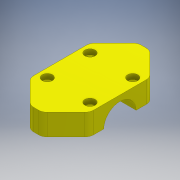
# Autodesk Inventor part: Y Carriage Clamp 1.0
Saved by Autodesk Inventor 2016 (Build 200138000, 138)
## iProperties
Created: 2017-02-14
Part Number: Y Carriage Clamp 1.0
Material: PC/ABS Plastic
Document SubType Name: Modeling
Designer: Scott
Density: 0.357273 g/cm^3
Appearance: Smooth - Yellow
Author: Scott
## iProperties of the stored document Y Carriage Clamp 1.0_3DPrint.ipt
Created: 2017-04-11
Part Number: Y Carriage Clamp 1.0_3DPrint
Material: Generic
Document SubType Name: Modeling
Designer: Scott
Density: 1 g/cm^3
Appearance: Default
Author: Scott
Autodesk Inventor part; units mm, degrees
ref_plane "YZ Plane" through (0, 0, 0) normal (1, 0, 0) x (0, 1, 0)
ref_plane "XZ Plane" through (0, 0, 0) normal (0, 1, 0) x (-1, 0, 0)
ref_plane "XY Plane" through (0, 0, 0) normal (0, 0, 1) x (1, 0, 0)
sketch "Sketch1" plane through (0, 0, 0) normal (0, 0, 1) x (1, 0, 0)
  line L0 (0, 0) -> (0, 37.7883) construction
  line L1 (0, 0) -> (33.2061, 0) construction
  line L2 (-17.5, 16.5) -> (17.5, 16.5)
  line L3 (17.5, 16.5) -> (17.5, -16.5)
  line L4 (17.5, -16.5) -> (-17.5, -16.5)
  line L5 (-17.5, -16.5) -> (-17.5, 16.5)
  line L6 (-17.5, 16.5) -> (-17.5, 17.5)
  line L7 (-17.5, 17.5) -> (-3.5, 31.5)
  line L8 (-3.5, 31.5) -> (3.5, 31.5)
  line L9 (3.5, 31.5) -> (17.5, 17.5)
  line L10 (17.5, 17.5) -> (17.5, 16.5)
  line L11 (-17.5, -16.5) -> (17.5, -16.5)
  line L12 (-17.5, -16.5) -> (-17.5, -17.5)
  line L13 (-17.5, -17.5) -> (-3.5, -31.5)
  line L14 (-3.5, -31.5) -> (3.5, -31.5)
  line L15 (3.5, -31.5) -> (17.5, -17.5)
  line L16 (17.5, -17.5) -> (17.5, -16.5)
  point P0 (0, 16.5)
  point P1 (17.5, 0)
  point P2 (0, -16.5)
  dimension "d0" = 35
  dimension "d1" = 33
  dimension "d2" = 1
  dimension "d3" = 1
  dimension "d4" = 45
  dimension "d5" = 45
  dimension "d6" = 31.5
  constraints: 34 end point, 5 symmetric about line, 3 parallel, 2 horizontal, 2 midpoint, 2 perpendicular, 2 point on line, 2 vertical
  measures "d0" distance of L2.start L2.end
  measures "d1" distance of L2.end L3.end
  measures "d2" distance from line of L2 L9.end
  measures "d3" distance of L2.start L6.end
  measures "d4" angle of L7 L2
  measures "d5" angle of L2 L9
  measures "d6" distance between parallel lines of L8 L1
extrude "Extrusion1" add sketch "Sketch1" along normal blind 12.5
sketch "Sketch2" plane through (17.5, -17.5, 0) normal (1, 0, 0) x (0, 0, -1)
  line L0 (0, 17.5) -> (18.5906, 17.5) construction
  circle A0 centre (0.25, 17.5) radius 9.5
  dimension "d9" = 0.25
  dimension "d10" = 19
  constraints: 2 end point, 1 centre point, 1 horizontal, 1 point on line
  measures "d9" distance of L0.start A0.centre
  measures "d10" diameter of A0
extrude "Extrusion2" cut sketch "Sketch2" against normal through all
sketch "Sketch3" plane through (0, 0, 12.5) normal (0, 0, 1) x (1, 0, 0)
  line L0 (0, 0) -> (23.8971, 0) construction
  line L1 (0, 0) -> (0, 42.5414) construction
  line L2 (-12.5, 12.5) -> (12.5, 12.5) construction
  line L3 (12.5, 12.5) -> (12.5, -12.5) construction
  line L4 (12.5, -12.5) -> (-12.5, -12.5) construction
  line L5 (-12.5, -12.5) -> (-12.5, 12.5) construction
  point P0 (12.5, 0)
  point P1 (0, 12.5)
  dimension "d13" = 25
  dimension "d14" = 25
  constraints: 12 end point, 4 coincident, 2 horizontal, 2 midpoint, 2 parallel, 2 point on line, 1 perpendicular, 1 vertical
  measures "d13" distance of L2.end L3.end
  measures "d14" distance of L2.start L2.end
hole "Hole1" at (-12.5, 12.5, 12.5) at (-12.5, -12.5, 12.5) at (12.5, -12.5, 12.5) at (12.5, 12.5, 12.5) direction (0, 0, -1) diameter 3.5 end through all counterbore diameter 6 counterbore depth 3
fillet "Fillet1" radius 5 8 edges at (3.5, 31.5, 6.25) (-3.5, 31.5, 6.25) (-17.5, 17.5, 6.25) (17.5, 17.5, 6.25) (-17.5, -17.5, 6.25) (-3.5, -31.5, 6.25) (3.5, -31.5, 6.25) (17.5, -17.5, 6.25)
sketch "Sketch4" plane through (0, 0, 0) normal (0, 0, -1) x (-1, 0, 0)
  line L0 (0, 0) -> (0, 38.8983) construction
  line L1 (0, 0) -> (0, -39.4176) construction
  circle A0 centre (0, 22.5) radius 5.5
  circle A1 centre (0, -22.5) radius 5.5
  dimension "d23" = 11
  dimension "d24" = 22.5
  dimension "d25" = 22.5
  constraints: 4 end point, 2 centre point, 2 point on line, 2 vertical, 1 equal radius
  measures "d23" diameter of A0
  measures "d24" distance of L0.start A0.centre
  measures "d25" distance of L0.start A1.centre
extrude "Extrusion3" cut sketch "Sketch4" against normal blind 5
sketch "Sketch5" plane through (-12.5, -12.5, 9.5) normal (0, 0, 1) x (1, 0, 0)
  circle A0 centre (0, 25) radius 1.75 projected
  circle A1 centre (0, 0) radius 1.75 projected
  circle A2 centre (25, 0) radius 1.75 projected
  circle A3 centre (25, 25) radius 1.75 projected
  point P0 (12.5, 12.5)
extrude "Extrusion4" add sketch "Sketch5" against normal blind 0.4
equation "\"d25\" = d24"
body "Solid1"
